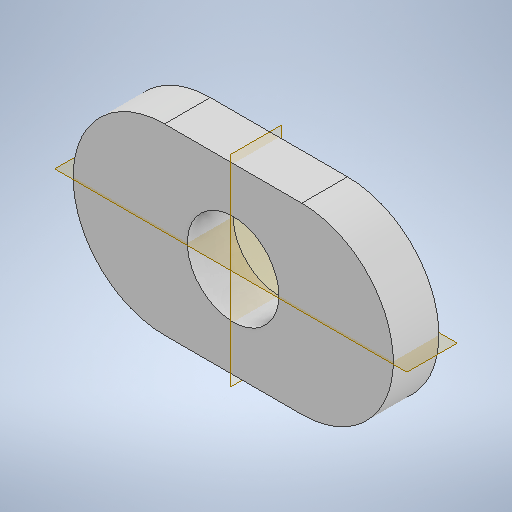
# Autodesk Inventor part: CS-Base
Saved by Autodesk Inventor 2025.1 (Build 291241000, 241)
## iProperties
Created: 2025-04-02
Part Number: CS-Base
Material: Generic
Document SubType Name: Modeling
Designer: a00584475
Density: 1 g/cm^3
Appearance: Default
Author: a00584475
Autodesk Inventor part; units mm, degrees
ref_plane "XY Plane" through (0, 0, 0) normal (0, 0, 1) x (1, 0, 0)
sketch "Sketch1" plane through (0, 0, 0) normal (0, 0, 1) x (1, 0, 0)
  point P0 (0, 0)
sketch "Sketch2" plane through (0, 0, 0) normal (0, 0, 1) x (1, 0, 0)
  line L0 (-9.525, 0) -> (9.525, 0) construction
  line L1 (-9.525, -12.7) -> (9.525, -12.7)
  line L2 (9.525, 12.7) -> (-9.525, 12.7)
  arc A0 (-9.525, 12.7) -> (-9.525, -12.7) centre (-9.525, 0) ccw
  arc A1 (9.525, -12.7) -> (9.525, 12.7) centre (9.525, 0) ccw
  circle A2 centre (0, 0) radius 6.35
  dimension "d0" = 9.525
  dimension "d1" = 25.4
  dimension "d2" = 12.7
  constraints: 8 end point, 4 point on circle, 4 tangent, 3 centre point, 1 coincident, 1 horizontal, 1 midpoint, 1 parallel
  measures "d0" distance of point (0, 0) L0.end
  measures "d1" diameter of A1
  measures "d2" diameter of A2
extrude "Extrusion1" add sketch "Sketch2" along normal blind 6.35
body "Solid1"
